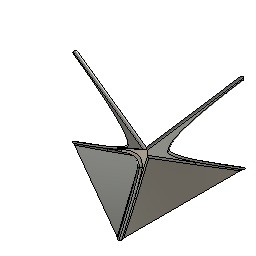
Static Stand Travel Case 2 v9 (Autodesk Fusion 360 archive; units mm, degrees)
design "Static Stand"
Autodesk Fusion 360 part; units mm, degrees
sketch "Sketch1" plane through (0, 0, 0) normal (0, 1, 0) x (1, 0, 0)
  line L0 (0, 0) -> (52.2558, 0)
  line L1 (52.2558, 0) -> (0, -73.9008)
  line L2 (0, -73.9008) -> (-104.5116, 0)
  line L3 (-104.5116, 0) -> (0, 0)
  line L4 (0, -73.9008) -> (0, 0) construction
  line L5 (0, -73.9008) -> (-128, -73.9008)
  line L6 (-128, -73.9008) -> (-128, 0)
  line L7 (-128, 0) -> (-104.5116, 0)
  line L8 (0, -73.9008) -> (128, -73.9008)
  line L9 (128, -73.9008) -> (128, 0)
  line L10 (128, 0) -> (52.2558, 0)
  line L11 (-104.5116, 0) -> (-84.0991, -14.4338)
  line L12 (-84.0991, -14.4338) -> (-25, -56.2232)
  line L13 (-25, -56.2232) -> (-25, -73.9008)
  spline S0 degree 3 poles (-104.5116, 0) (-84.0991, -14.4338) (-25, -56.2232) (-25, -73.9008) knots 0 0 0 0 1 1 1 1
  line L14 (104.5116, 0) -> (-104.5116, -147.8017)
  spline S1 degree 3 poles (-104.5116, -147.8017) (-84.0991, -133.3679) (-25, -91.5785) (-25, -73.9008) knots 0 0 0 0 1 1 1 1
  line L15 (-104.5116, -147.8017) -> (-84.0991, -133.3679)
  line L16 (-84.0991, -133.3679) -> (-25, -91.5785)
  line L17 (-25, -91.5785) -> (-25, -73.9008)
  line L18 (0, -78.7998) -> (-102.2022, -151.0677)
  line L19 (-104.5116, -147.8017) -> (-102.2022, -151.0677)
  line L20 (0, -73.9008) -> (0, -78.7998)
  dimension "d2" = 52.2558
  dimension "d3" = 90.5097
  dimension "d4" = 73.9008
  dimension "d5" = 90
  dimension "d6" = 128
  dimension "d7" = 128
  dimension "d14" = 25
  dimension "d19" = 25
  dimension "d21" = 4
  constraint coincident L0.start L3.end
  constraint horizontal L0
  constraint parallel L0 L3
  constraint vertical L4
  constraint perpendicular L4 L5
  constraint perpendicular L5 L6
  constraint horizontal L7
  constraint perpendicular L4 L8
  constraint perpendicular L8 L9
  constraint horizontal L10
  constraint coincident L5 L13.end
  constraint coincident L2 L11.end
  constraint coincident L2 L12.end
  constraint vertical L13
  constraint symmetric L1.end L5 L2.start
  constraint symmetric L2.end L5 L14.end
  constraint symmetric L5 L13.end S0.end
  constraint symmetric L5 S0 S1
  constraint perpendicular L5 L20
  constraint parallel L14 L18
  constraint perpendicular L18 L19
  constraint coincident L1.end L14
  measures "d2" distance of L0.start L0.end
  measures "d3" distance of L0.end L1.end
  measures "d4" distance of L1.end L0.start
  measures "d5" angle of L1 L2
  measures "d6" distance of L1.end L5.end
  measures "d7" distance of L1.end L8.end
  measures "d14" distance of L1.end L13.end
  measures "d19" distance of L2.end L11.end
  measures "d21" distance of L14.end L18.end
extrude "Extrude1" add sketch "Sketch1" along normal mid plane 256 contours L0 L1 L2 L3 L11 L12 | L5 L6 L7 S0 | L2 L11 L12 L13 S0 | L2 L5 L13 makes body 1
extrude "Extrude3" add sketch "Sketch1" along normal mid plane 5 separate body contours L14 S1 L15 L16 L17 | L0 L1 L2 L3 L11 L12 | L2 L11 L12 L13 S0 | L2 L5 L13 | L5 L14 L17 | L14 L15 L16 L18 L19 L20 makes body 2
sketch "Sketch2" plane through (-139.3487, 0, 98.5344) normal (-0.816497, 0, 0.57735) x (0, -1, 0)
  line L0 (2.5, 64.3398) -> (-2.5, 64.3398)
  line L1 (-2.5, 64.3398) -> (-2.5, 60.3398)
  line L2 (-2.5, 60.3398) -> (2.5, 60.3398)
  line L3 (2.5, 60.3398) -> (2.5, 64.3398)
  line L4 (-2.5, 64.3398) -> (0, 66.8398) construction
  line L5 (-2.5, 64.3398) -> (1.1605, 64.3398) construction
  line L6 (0, 60.3398) -> (0, 134.2406) construction
  arc A0 (-2.5, 64.3398) -> (2.5, 64.3398) centre (0, 66.8398) ccw
  dimension "d24" = 45
  constraint horizontal L5
  constraint coincident L0.end L1.start
  constraint coincident L4.end L6
  constraint coincident L4.end A0.centre
  measures "d24" angle of L4 L5
extrude "Extrude4" cut sketch "Sketch2" against normal through all contours L0 A0 bodies 2
fillet "Fillet1" radius 2.5 4 edges at (-57.1011, -2.5, 112.0677) (-57.1011, -2.5, 35.7339) (-57.1011, 2.5, 35.7339) (-57.1011, 2.5, 112.0677) on bodies 2
fillet "Fillet2" radius 2.5 4 edges at (-102.6352, -2.5, 150.4553) (-104.0884, -1.7686, 148.4002) (-104.0893, 1.767, 148.3989) (-102.6352, 2.5, 150.4553) on bodies 2
copy_body "CopyPasteBodies1" bodies 1 makes body 3
move_body "Move1" bodies 3 to x (-0.5, -0.866025, 0) y (0.866025, -0.5, 0) z (0, 0, 1) at (0, 0, 0)
copy_body "CopyPasteBodies2" bodies 3 makes body 4
move_body "Move2" bodies 4 to x (-0.5, -0.866025, 0) y (0.866025, -0.5, 0) z (0, 0, 1) at (0, 0, 0)
combine "Combine1" operation intersect target body 1 tool bodies 3
combine "Combine2" operation intersect target body 1 tool bodies 4
ref_plane "WorkPlane1" through (0, 0, 73.9008) normal (0, 0, 1) x (1, 0, 0)
copy_body "CopyPasteBodies3" bodies 2 makes body 5
move_body "Move3" bodies 5 to x (-0.5, -0.866025, 0) y (0.866025, -0.5, 0) z (0, 0, 1) at (0, 0, 0)
copy_body "CopyPasteBodies4" bodies 5 makes body 6
move_body "Move4" bodies 6 to x (-0.5, -0.866025, 0) y (0.866025, -0.5, 0) z (0, 0, 1) at (0, 0, 0)
shell "Shell2" thickness 5 removed faces 1 at (0, 0, 0) on bodies 1
combine "Combine3" operation add target body 1 tool bodies 6 5 2
fillet "Fillet4" radius 5 6 edges at (27.5713, -42.7548, 34.9092) (27.5713, 42.7548, 34.9092) (-50.8124, 2.5, 34.9092) (23.2411, 45.2548, 34.9092) (23.2411, -45.2548, 34.9092) (-50.8124, -2.5, 34.9092) on bodies 1
split "Split1" by plane through (0, 0, 73.9008) normal (0, 0, 1) bodies 1 makes body 7 at (-34.6037, -2.2461, 102.9862)
scale "Scale1" factors (1, 1, 0.5) about (0, 0, 73.9008) bodies 1
combine "Combine4" operation add target body 1 tool bodies 7
equation "side = 128 mm"
equation "d2 = side * sqrt(1 / 6)"
equation "d3 = side * sqrt(1 / 2)"
equation "d6 = side"
equation "d7 = side"
equation "d8 = side"
equation "center_radius = 25 mm"
equation "d14 = center_radius"
